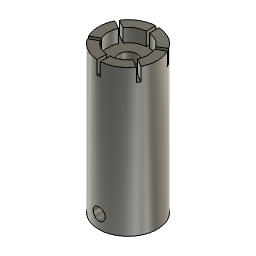
Amazon wheel axel (Autodesk Fusion 360 design; units mm, degrees)
Autodesk Fusion 360 part; units mm, degrees
sketch "Skizze1" plane through (0, 0, 0) normal (0, 0, 1) x (1, 0, 0)
  circle A0 centre (0, 0) radius 13.25
  dimension "d1" = 26.5
  constraint coincident A0.centre origin
  measures "d1" diameter of A0
extrude "Extrusion1" add sketch "Skizze1" along normal blind 66
sketch "Skizze2" plane through (0, 0, 66) normal (0, 0, 1) x (-1, 0, 0)
  circle A0 centre (0, 0) radius 13.25
  circle A1 centre (0, 0) radius 9
  line L0 (0.75, -14.5) -> (-0.75, -14.5)
  line L1 (-0.75, -14.5) -> (-0.75, -8.5)
  line L2 (-0.75, -8.5) -> (0.75, -8.5)
  line L3 (0.75, -8.5) -> (0.75, -14.5)
  line L4 (12.1824, -7.8995) -> (6.9862, -4.8995)
  line L5 (12.9324, -6.6005) -> (12.1824, -7.8995)
  line L6 (7.7362, -3.6005) -> (12.9324, -6.6005)
  line L7 (6.9862, -4.8995) -> (7.7362, -3.6005)
  line L8 (12.9324, 6.6005) -> (7.7362, 3.6005)
  line L9 (12.1824, 7.8995) -> (12.9324, 6.6005)
  line L10 (6.9862, 4.8995) -> (12.1824, 7.8995)
  line L11 (7.7362, 3.6005) -> (6.9862, 4.8995)
  line L12 (0.75, 14.5) -> (0.75, 8.5)
  line L13 (-0.75, 14.5) -> (0.75, 14.5)
  line L14 (-0.75, 8.5) -> (-0.75, 14.5)
  line L15 (0.75, 8.5) -> (-0.75, 8.5)
  line L16 (-12.1824, 7.8995) -> (-6.9862, 4.8995)
  line L17 (-12.9324, 6.6005) -> (-12.1824, 7.8995)
  line L18 (-7.7362, 3.6005) -> (-12.9324, 6.6005)
  line L19 (-6.9862, 4.8995) -> (-7.7362, 3.6005)
  line L20 (-12.9324, -6.6005) -> (-7.7362, -3.6005)
  line L21 (-12.1824, -7.8995) -> (-12.9324, -6.6005)
  line L22 (-6.9862, -4.8995) -> (-12.1824, -7.8995)
  line L23 (-7.7362, -3.6005) -> (-6.9862, -4.8995)
  dimension "d4" = 18
  dimension "d5" = 1.5
  dimension "d6" = 6
  dimension "d7" = 0.75
  dimension "d8" = 8.5
  dimension "d10" = 360
  constraint coincident A0.centre A1.centre
  constraint horizontal L0
  constraint vertical L1
  constraint horizontal L2
  constraint vertical L3
  measures "d4" diameter of A1
  measures "d5" distance of L0.start L0.end
  measures "d6" distance of L0.start L2.end
  measures "d7" horizontal distance of A0.centre L0.start
  measures "d8" vertical distance of A0.centre L2.end
extrude "Extrusion2" cut sketch "Skizze2" against normal blind 6 contours A0 A1 L8 L10 | A0 A1 L4 L6 | A1 L8 L10 L11 | A1 L1 L2 L3 L4 L6 L7 L8 L10 L11 L12 L14 L15 L16 L18 L19 L20 L22 L23 | A1 L4 L6 L7 | A0 A1 L12 L14 | A0 A1 L1 L3 | A1 L12 L14 L15 | A1 L1 L2 L3 | A0 A1 L16 L18 | A0 A1 L20 L22 | A1 L16 L18 L19 | A1 L20 L22 L23
sketch "Skizze3" plane through (0, 0, 60) normal (0, 0, 1) x (-1, 0, 0)
  arc A0 (-11.8314, -5.9649) -> (-11.0814, -7.2639) centre (0, 0) ccw
  line L0 (-11.0814, -7.2639) -> (-7.3921, -5.1339)
  arc A1 (-7.3921, -5.1339) -> (-0.75, -8.9687) centre (0, 0) ccw
  line L1 (-0.75, -8.9687) -> (-0.75, -13.2288)
  arc A2 (-0.75, -13.2288) -> (0.75, -13.2288) centre (0, 0) ccw
  line L2 (0.75, -13.2288) -> (0.75, -8.9687)
  arc A3 (0.75, -8.9687) -> (7.3921, -5.1339) centre (0, 0) ccw
  line L3 (7.3921, -5.1339) -> (11.0814, -7.2639)
  arc A4 (11.0814, -7.2639) -> (11.8314, -5.9649) centre (0, 0) ccw
  line L4 (11.8314, -5.9649) -> (8.1421, -3.8348)
  arc A5 (8.1421, -3.8348) -> (8.1421, 3.8348) centre (0, 0) ccw
  line L5 (8.1421, 3.8348) -> (11.8314, 5.9649)
  arc A6 (11.8314, 5.9649) -> (11.0814, 7.2639) centre (0, 0) ccw
  line L6 (11.0814, 7.2639) -> (7.3921, 5.1339)
  arc A7 (7.3921, 5.1339) -> (0.75, 8.9687) centre (0, 0) ccw
  line L7 (0.75, 8.9687) -> (0.75, 13.2288)
  arc A8 (0.75, 13.2288) -> (-0.75, 13.2288) centre (0, 0) ccw
  line L8 (-0.75, 13.2288) -> (-0.75, 8.9687)
  arc A9 (-0.75, 8.9687) -> (-7.3921, 5.1339) centre (0, 0) ccw
  line L9 (-7.3921, 5.1339) -> (-11.0814, 7.2639)
  arc A10 (-11.0814, 7.2639) -> (-11.8314, 5.9649) centre (0, 0) ccw
  line L10 (-11.8314, 5.9649) -> (-8.1421, 3.8348)
  arc A11 (-8.1421, 3.8348) -> (-8.1421, -3.8348) centre (0, 0) ccw
  line L11 (-8.1421, -3.8348) -> (-11.8314, -5.9649)
  circle A12 centre (0, 0) radius 4
  dimension "d13" = 8
  constraint concentric A0 A12
  measures "d13" diameter of A12
extrude "Extrusion3" cut sketch "Skizze3" against normal blind 15 contours A12
sketch "Skizze4" plane through (0, 0, 0) normal (0, 0, -1) x (1, 0, 0)
  circle A0 centre (0, 0) radius 13.25
  circle A1 centre (0, 0) radius 3
  line L0 (-1.6583, 2.5) -> (1.6583, 2.5)
  dimension "d16" = 6
  dimension "d17" = 2.5
  constraint coincident A0.centre A1.centre
  constraint coincident A1 L0.start
  constraint coincident A1 L0.end
  constraint horizontal L0
  measures "d16" diameter of A1
  measures "d17" vertical distance of A0.centre L0.start
extrude "Extrusion4" cut sketch "Skizze4" against normal blind 12 contours A1 L0 picked at (0.6261, 0.5577)
sketch "Skizze5" plane through (0, -2.5, 0) normal (0, 1, 0) x (-1, 0, 0)
  line L0 (-1.6583, 0) -> (1.6583, 0)
  line L1 (1.6583, 0) -> (1.6583, 12)
  line L2 (1.6583, 12) -> (-1.6583, 12)
  line L3 (-1.6583, 12) -> (-1.6583, 0)
  circle A0 centre (0, 6) radius 2.75
  dimension "d20" = 5.5
  dimension "d21" = 6
  measures "d20" diameter of A0
  measures "d21" distance of origin A0.centre
extrude "Extrusion5" cut sketch "Skizze5" along normal blind 3 contours L3 A0 | L1 L3 A0 | L1 A0
sketch "Skizze6" plane through (0, -2.5, 0) normal (0, 1, 0) x (-1, 0, 0)
  line L0 (1.6583, 8.1937) -> (1.6583, 12)
  line L1 (1.6583, 12) -> (-1.6583, 12)
  line L2 (-1.6583, 12) -> (-1.6583, 8.1937)
  arc A0 (-1.6583, 8.1937) -> (-1.6583, 3.8063) centre (0, 6) ccw
  line L3 (-1.6583, 3.8063) -> (-1.6583, 0)
  line L4 (-1.6583, 0) -> (1.6583, 0)
  line L5 (1.6583, 0) -> (1.6583, 3.8063)
  arc A1 (1.6583, 3.8063) -> (1.6583, 8.1937) centre (0, 6) ccw
  circle A2 centre (0, 6) radius 2.75
  dimension "d24" = 5.5
  constraint concentric A0 A2
  measures "d24" diameter of A2
extrude "Extrusion6" cut sketch "Skizze6" against normal blind 15 contours A0 A1 A2
